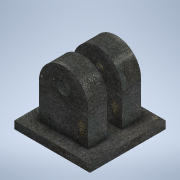
# Autodesk Inventor part: 03_10 soporte02
Saved by Autodesk Inventor 2021 (Build 250183000, 183)
## iProperties
Created: 2021-06-25
Part Number: 03_10 soporte02
Material: Acero ASTM A36
Document SubType Name: Modeling
Designer: Almanzor
Density: 7.85 g/cm^3
Appearance: Placa
Author: Almanzor
Autodesk Inventor part; units mm, degrees
ref_plane "YZ Plane" through (0, 0, 0) normal (1, 0, 0) x (0, 1, 0)
ref_plane "XZ Plane" through (0, 0, 0) normal (0, 1, 0) x (-1, 0, 0)
ref_plane "XY Plane" through (0, 0, 0) normal (0, 0, 1) x (1, 0, 0)
sketch "Boceto1" plane through (0, 0, 0) normal (0, 1, 0) x (-1, 0, 0)
  line L0 (50, 50) -> (-50, 50)
  line L1 (-50, 50) -> (-50, -50)
  line L2 (-50, -50) -> (50, -50)
  line L3 (50, -50) -> (50, 50)
  line L4 (50, 50) -> (-50, -50) construction
  line L5 (-50, 50) -> (50, -50) construction
  point P0 (0, 0)
  dimension "d0" = 100
  dimension "d1" = 100
  constraints: 12 end point, 2 midpoint, 2 parallel, 1 horizontal, 1 perpendicular
  measures "d0" distance of L1.end L2.end
  measures "d1" distance of L0.end L1.end
extrude "Extrusión1" add sketch "Boceto1" along normal blind 10
sketch "Boceto2" plane through (0, 10, 0) normal (0, 1, 0) x (1, 0, 0)
  line L0 (32.5, -35) -> (-32.5, -35)
  line L1 (-32.5, -35) -> (-32.5, -10)
  line L2 (-32.5, -10) -> (32.5, -10)
  line L3 (32.5, -10) -> (32.5, -35)
  line L4 (0, 0) -> (-40.0762, 0)
  line L5 (32.5, 35) -> (-32.5, 35)
  line L6 (-32.5, 35) -> (-32.5, 10)
  line L7 (-32.5, 10) -> (32.5, 10)
  line L8 (32.5, 10) -> (32.5, 35)
  dimension "d4" = 25
  dimension "d5" = 65
  dimension "d6" = 10
  dimension "d7" = 32.5
  dimension "d8" = 10
  constraints: 18 end point, 4 symmetric about line, 2 horizontal, 2 parallel, 1 perpendicular
  measures "d4" distance of L0.end L1.end
  measures "d5" distance of L0.start L0.end
  measures "d6" distance from line of L4.start L2
  measures "d7" distance from line of L4.start L1
  measures "d8" distance from line of L4.start L7
extrude "Extrusión2" add sketch "Boceto2" along normal blind 80
sketch "Boceto3" plane through (-32.5, 10, 35) normal (0, 0, 1) x (1, 0, 0)
  circle A0 centre (32.5, 55) radius 8.5
  line L0 (0, 0) -> (0, 80) projected
  line L1 (0, 80) -> (65, 80) projected
  point P0 (32.5, -10)
  dimension "d11" = 17
  dimension "d12" = 32.5
  dimension "d13" = 25
  constraints: 1 centre point
  measures "d11" diameter of A0
  measures "d12" distance from line of L0 A0.centre
  measures "d13" distance from line of L1 A0.centre
extrude "Extrusión3" cut sketch "Boceto3" against normal blind 80
fillet "Empalme1" radius 32.5 4 edges at (-32.5, 90, 22.5) (32.5, 90, 22.5) (32.5, 90, -22.5) (-32.5, 90, -22.5)
